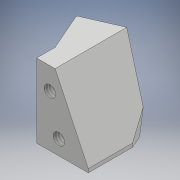
# Autodesk Inventor part: CMC extension endstop
Saved by Autodesk Inventor 2017 (Build 210142000, 142)
## iProperties
Created: 2018-02-12
Part Number: CMC extension endstop
Material: Generic
Document SubType Name: Modeling
Designer: JT
Density: 1 g/cm^3
Appearance: Default
Author: JT
Autodesk Inventor part; units mm, degrees
ref_plane "YZ Plane" through (0, 0, 0) normal (1, 0, 0) x (0, 1, 0)
ref_plane "XZ Plane" through (0, 0, 0) normal (0, 1, 0) x (-1, 0, 0)
ref_plane "XY Plane" through (0, 0, 0) normal (0, 0, 1) x (1, 0, 0)
sketch "Sketch1" plane through (0, 0, 0) normal (0, 0, 1) x (1, 0, 0)
  line L0 (0, 0) -> (0, 2.5)
  line L1 (0, 2.5) -> (-2.2441, 7.6403)
  line L2 (-2.2441, 7.6403) -> (4.9187, 10.7674)
  line L3 (4.9187, 10.7674) -> (7, 6)
  line L4 (7, 6) -> (7, 0)
  line L5 (7, 0) -> (0, 0)
  dimension "d5" = 23.584
  dimension "d6" = 2.5
  dimension "d7" = 7
  dimension "d9" = 6
  dimension "d14" = 7.9
  constraints: 12 end point, 2 parallel, 2 perpendicular, 1 vertical
  measures "d5" angle of L4 L3
  measures "d6" distance of L0.start L0.end
  measures "d7" distance of L4.end L0.start
  measures "d9" distance of L4.end L3.end
  measures "d14" distance from line of L0.start L2
extrude "Extrusion1" add sketch "Sketch1" along normal blind 10
sketch "Sketch2" plane through (6.9048, 6.218, 0) normal (-0.916472, -0.4000988, 0) x (0, 0, 1)
  line L0 (0, 4.964) -> (10, 4.964) projected
  line L1 (10, 4.964) -> (10, -0.6448) projected
  line L2 (10, 4.964) -> (0, 1.618)
  line L3 (0, 1.618) -> (0, 4.964)
  point P0 (0, -2.936)
  dimension "d2" = 18.5
  constraints: 4 end point, 1 vertical
  measures "d2" angle of L2 L0
extrude "Extrusion2" cut sketch "Sketch2" along normal through all both and the other way through all
sketch "Sketch3" plane through (0, 0, 0) normal (0, -1, 0) x (1, 0, 0)
  line L0 (7, 0) -> (0, 0) projected
  line L1 (7, 0) -> (7, 10) projected
  line L2 (0, 10) -> (7, 10) projected
  line L3 (0, 0) -> (0, 10) projected
  line L4 (2.5, 10) -> (7, 0.5)
  dimension "d12" = 2.5
  dimension "d13" = 0.5
  constraints: 2 end point, 2 point on line
  measures "d12" distance of L2.start L4.start
  measures "d13" distance from line of L0 L4.end
extrude "Extrusion3" cut sketch "Sketch3" against normal through all contours L4 L2 L1
sketch "Sketch4" plane through (0, 0, 0) normal (0, -1, 0) x (1, 0, 0)
  point P0 (0, 0)
  point P1 (3, 2)
  point P2 (1.8, 7)
  dimension "d22" = 3
  dimension "d23" = 2
  dimension "d24" = 7
  dimension "d25" = 1.8
  measures "d22" horizontal distance of point (3, 2) point (0, 0)
  measures "d23" vertical distance of point (0, 0) point (3, 2)
  measures "d24" vertical distance of point (1.8, 7) point (0, 0)
  measures "d25" horizontal distance of point (0, 0) point (1.8, 7)
hole "Hole1" at (3, 0, 2) at (1.8, 0, 7) direction (0, 1, 0) diameter 1.567 depth 5 tip angle 118 thread size "M2x0.4" class "6H" standard "ANSI Metric M Profile"
equation "\"d5\" = thumb_axis_beta_local"
equation "\"thumb_axis_beta_local\" = thumb_axis_beta"
body "Solid1"
